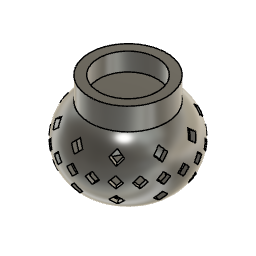
Kertastjaki v5 (Autodesk Fusion 360 design; units mm, degrees)
Autodesk Fusion 360 part; units mm, degrees
sketch "Sketch6" plane through (0, 0, 0) normal (0, 0, 1) x (1, 0, 0)
  circle A0 centre (0, 0) radius 27.5
  dimension "d16" = 55
  constraint coincident A0.centre origin
  measures "d16" diameter of A0
extrude "Extrude4" add sketch "Sketch6" along normal blind 3
sketch "Sketch7" plane through (0, 0, 3) normal (0, 0, 1) x (-1, 0, 0)
  circle A0 centre (0, 0) radius 27.5
  circle A1 centre (0, 0) radius 21
  circle A2 centre (0, 0) radius 27.5
  dimension "d19" = 42
  dimension "d20" = 55
  constraint coincident A0.centre A1.centre
  measures "d19" diameter of A1
  measures "d20" diameter of A2
extrude "Extrude5" add sketch "Sketch7" along normal blind 13
sketch "Sketch8" plane through (0, 0, 0) normal (0, 1, 0) x (1, 0, 0)
  line L0 (0, 0) -> (0, 50)
  line L1 (0, 0) -> (27.5, 0)
  line L2 (0, 50) -> (20, 50)
  arc A0 (27.5, 0) -> (20, 50) centre (12.2794, 23.2794) ccw
  arc A1 (25.8583, 2.5109) -> (19.1673, 47.1179) centre (12.2794, 23.2794) ccw
  line L3 (25.8583, 2.5109) -> (22.0179, 0)
  line L4 (19.1673, 47.1179) -> (0, 47.1179)
  dimension "d23" = 50
  dimension "d24" = 27.5
  dimension "d25" = 20
  dimension "d26" = -3
  constraint coincident L0.start L1.start
  constraint vertical L0
  constraint perpendicular L0 L1
  constraint perpendicular L0 L2
  constraint coincident L1 L3.end
  constraint tangent A1 L3
  constraint coincident L0 L4.end
  constraint perpendicular L0 L4
  measures "d23" distance of L0.start L0.end
  measures "d24" distance of L0.start L1.end
  measures "d25" distance of L0.end L2.end
revolve "Revolve1" add sketch "Sketch8" angle 360 about axis through (0, 0, 1.75) along (0, 0, 1) contours L0 L1 L2 A0 A1 L3 L4
sketch "Sketch9" plane through (0, 0, 0) normal (0, 1, 0) x (1, 0, 0)
  line L0 (0, 0) -> (0, 23)
  line L1 (0, 23) -> (4, 23)
  line L2 (0, 23) -> (0, 27)
  line L3 (0, 23) -> (0, 19)
  line L4 (0, 27) -> (4, 23)
  line L5 (0, 19) -> (4, 23)
  line L6 (0, 27) -> (-4, 23)
  line L7 (0, 19) -> (-4, 23)
  dimension "d28" = 23
  dimension "d29" = 4
  dimension "d30" = 4
  dimension "d31" = 4
  constraint coincident L0.start origin
  constraint vertical L0
  constraint perpendicular L0 L1
  constraint perpendicular L1 L2
  constraint perpendicular L1 L3
  constraint symmetric L0 L1.end L6.end
  constraint symmetric L0 L2.end L4.start
  constraint symmetric L0 L3.end L5.start
  measures "d28" distance of L0.start L0.end
  measures "d29" distance of L0.end L1.end
  measures "d30" distance of L0.end L2.end
  measures "d31" distance of L0.end L3.end
extrude "Extrude6" cut sketch "Sketch9" against normal blind 50
pattern_circular "C-Pattern1" count 20 over 360 about axis through (0, 0, 1.75) along (0, 0, 1) of "Extrude6"
sketch "Sketch10" plane through (0, 0, 0) normal (0, 1, 0) x (1, 0, 0)
  line L0 (0, 0) -> (0, 10)
  line L1 (0, 50) -> (0, 36)
  line L2 (0, 10) -> (0, 14)
  line L3 (0, 10) -> (0, 6)
  line L4 (0, 10) -> (4, 10)
  line L5 (4, 10) -> (0, 6)
  line L6 (4, 10) -> (0, 14)
  line L7 (0, 36) -> (0, 32)
  line L8 (0, 36) -> (0, 40)
  line L9 (0, 36) -> (4, 36)
  line L10 (0, 32) -> (4, 36)
  line L11 (0, 40) -> (4, 36)
  line L12 (-4, 10) -> (0, 6)
  line L13 (-4, 10) -> (0, 14)
  line L14 (0, 32) -> (-4, 36)
  line L15 (0, 40) -> (-4, 36)
  dimension "d39" = 10
  dimension "d40" = 14
  dimension "d41" = 4
  dimension "d42" = 4
  dimension "d43" = 4
  dimension "d44" = 4
  dimension "d45" = 4
  dimension "d46" = 4
  constraint coincident L0.start origin
  constraint vertical L0
  constraint vertical L1
  constraint parallel L0 L2
  constraint parallel L0 L3
  constraint perpendicular L3 L4
  constraint parallel L1 L7
  constraint parallel L1 L8
  constraint perpendicular L1 L9
  constraint symmetric L0 L2.end L6.end
  constraint symmetric L0 L3.end L5.end
  constraint symmetric L0 L4.end L12.start
  constraint symmetric L0 L7.end L10.start
  constraint symmetric L0 L8.end L11.start
  constraint symmetric L0 L9.end L14.end
  measures "d39" distance of L0.start L0.end
  measures "d40" distance of L1.start L1.end
  measures "d41" distance of L0.end L2.end
  measures "d42" distance of L0.end L3.end
  measures "d43" distance of L0.end L4.end
  measures "d44" distance of L1.end L7.end
  measures "d45" distance of L1.end L8.end
  measures "d46" distance of L1.end L9.end
extrude "Extrude8" cut sketch "Sketch10" along normal blind 50
pattern_circular "C-Pattern3" count 10 over 360 about axis through (0, 0, 1.75) along (0, 0, 1) of "Extrude8"
